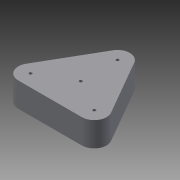
# Autodesk Inventor part: RollerMounter
Saved by Autodesk Inventor 2013 (Build 170138000, 138)
## iProperties
Created: 2013-08-11
Part Number: RollerMounter
Material: Generic
Document SubType Name: Modeling
Designer: dkboone
Density: 1 g/cm^3
Author: dkboone
Autodesk Inventor part; units mm, degrees
ref_plane "YZ Plane" through (0, 0, 0) normal (1, 0, 0) x (0, 1, 0)
ref_plane "XZ Plane" through (0, 0, 0) normal (0, 1, 0) x (-1, 0, 0)
ref_plane "XY Plane" through (0, 0, 0) normal (0, 0, 1) x (1, 0, 0)
sketch "Sketch1" plane through (0, 0, 0) normal (0, 1, 0) x (-1, 0, 0)
  line L0 (-8.255, 7.149) -> (8.255, 7.149) construction
  line L1 (8.255, 7.149) -> (0, -7.149) construction
  line L2 (0, -7.149) -> (-8.255, 7.149) construction
  line L3 (0, -7.149) -> (0, 7.149) construction
  circle A0 centre (-8.255, 7.149) radius 1.524 construction
  circle A1 centre (8.255, 7.149) radius 1.524 construction
  circle A2 centre (0, -7.149) radius 1.524 construction
  circle A3 centre (-8.255, 7.149) radius 0.381
  circle A4 centre (8.255, 7.149) radius 0.381
  circle A5 centre (0, -7.149) radius 0.381
  line L4 (-8.255, 10.324) -> (8.255, 10.324)
  line L5 (-11.0046, 5.5615) -> (-2.7496, -8.7365)
  line L6 (11.0046, 5.5615) -> (2.7496, -8.7365)
  arc A6 (-8.255, 10.324) -> (-11.0046, 5.5615) centre (-8.255, 7.149) ccw
  arc A7 (11.0046, 5.5615) -> (8.255, 10.324) centre (8.255, 7.149) ccw
  arc A8 (-2.7496, -8.7365) -> (2.7496, -8.7365) centre (0, -7.149) ccw
  line L7 (8.255, 7.149) -> (-4.1275, 0) construction
  line L8 (-8.255, 7.149) -> (4.1275, 0) construction
  circle A9 centre (0, 2.383) radius 0.381
  point P0 (0, 0)
  point P1 (0, 0)
  dimension "d1" = 16.51
  dimension "d2" = 3.048
  dimension "d3" = 0.762
  dimension "d4" = 3.175
  dimension "d5" = 0.762
  constraints: 18 end point, 10 centre point, 7 coincident, 6 point on circle, 6 tangent, 4 equal radius, 4 midpoint, 3 concentric, 2 parallel, 2 point on line, 1 equal length, 1 horizontal, 1 perpendicular, 1 vertical
  measures "d1" distance of L0.start L0.end
  measures "d2" diameter of A0
  measures "d3" diameter of A3
  measures "d4" radius of A6
  measures "d5" diameter of A9
extrude "Extrusion1" add sketch "Sketch1" along normal blind 6.35
body "Solid1"
